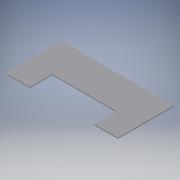
# Autodesk Inventor part: Pared sur
Saved by Autodesk Inventor 2016 (Build 200138000, 138)
## iProperties
Created: 2015-11-12
Part Number: Pared sur
Material: Generic
Document SubType Name: Modeling
Designer: serge
Density: 1 g/cm^3
Mass: 1.9558e+06 g
Surface Area: 787272 cm^2
Volume: 1.9558e+06 cm^3
Appearance: Valor por defecto
Author: serge
Autodesk Inventor part; units mm, degrees
ref_plane "YZ Plane" through (0, 0, 0) normal (1, 0, 0) x (0, 1, 0)
ref_plane "XZ Plane" through (0, 0, 0) normal (0, 1, 0) x (-1, 0, 0)
ref_plane "XY Plane" through (0, 0, 0) normal (0, 0, 1) x (1, 0, 0)
sketch "Sketch1" plane through (0, 0, 0) normal (0, 0, 1) x (1, 0, 0)
  line L0 (-4279.0972, -2988.6181) -> (20.9028, -2988.6181)
  line L1 (20.9028, -2988.6181) -> (20.9028, 11.3819)
  line L2 (20.9028, 11.3819) -> (-4279.0972, 11.3819)
  line L3 (-4279.0972, 11.3819) -> (-4279.0972, -2988.6181)
  point P0 (0, 0)
  dimension "Ancho" = 4300
  dimension "Alto" = 3000
  constraints: 8 end point, 2 parallel, 1 horizontal, 1 perpendicular
  measures "Ancho" distance of L1.end L2.end
  measures "Alto" distance of L0.end L1.end
extrude "Extrusion1" add sketch "Sketch1" along normal blind 50.8
sketch "Sketch2" plane through (0, 0, 50.8) normal (0, 0, 1) x (1, 0, 0)
  line L0 (-4279.0972, -2988.6181) -> (20.9028, -2988.6181) projected
  line L1 (-3579.0972, -988.6181) -> (-679.0972, -988.6181)
  line L2 (-679.0972, -988.6181) -> (-679.0972, -2988.6181)
  line L3 (-679.0972, -2988.6181) -> (-3579.0972, -2988.6181)
  line L4 (-3579.0972, -2988.6181) -> (-3579.0972, -988.6181)
  line L5 (-3579.0972, -988.6181) -> (-679.0972, -2988.6181) construction
  line L6 (-679.0972, -988.6181) -> (-3579.0972, -2988.6181) construction
  line L7 (-4279.0972, 11.3819) -> (-4279.0972, -2988.6181) projected
  point P0 (0, 0)
  point P1 (-2129.0972, -1988.6181)
  dimension "Distanciapuerta" = 2900
  dimension "Alturapuerta" = 2000
  dimension "d10" = 700
  constraints: 12 end point, 2 midpoint, 2 parallel, 1 horizontal, 1 perpendicular, 1 point on line
  measures "Distanciapuerta" distance of L1.start L1.end
  measures "Alturapuerta" distance of L1.end L2.end
  measures "d10" distance between parallel lines of L7 L4
extrude "Extrusion2" cut sketch "Sketch2" against normal through all
equation "\"Ancho\" = PL_S"
equation "\"Alto\" = PA_S"
equation "\"Espesor\" = PE_S"
equation "\"Distanciapuerta\" = DP_S"
equation "\"Alturapuerta\" = AP_S"
equation "\"d10\" = -0.5 * DP_S + 0.5 * PL_S"
equation "\"PL_S\" = 4300"
equation "\"PA_S\" = 3000"
equation "\"PE_S\" = 50.8"
equation "\"DP_S\" = 2900"
equation "\"AP_S\" = 2000"
equation "\"PE_N\" = 50.8"
equation "\"PE_EO\" = 50.8"
equation "\"T_E\" = 50.8"
equation "\"lon_ve\" = 512.5"
equation "\"n_a\" = 3"
equation "\"t_a\" = 19.05"
equation "\"d_a\" = 128.125"
equation "\"lon_ho\" = 749"
equation "\"d_bor\" = 59.92"
equation "\"lon_gui\" = 187.25"
equation "\"esp_gui\" = 461.25"
equation "\"lon_ve2\" = 498.475"
equation "\"n_a2\" = 3"
equation "\"t_a2\" = 124.61875"
equation "\"d_a2\" = 124.61875"
equation "\"lon_ho2\" = 933.45"
equation "\"d_bor2\" = 74.676"
equation "\"lon_gui2\" = 233.3625"
equation "\"esp_gui2\" = 448.6275"
equation "\"UE_L\" = 2111"
equation "\"UE_A\" = 1025"
equation "\"UE_AN\" = 749"
equation "\"UC_L\" = 1314.45"
equation "\"UC_A\" = 996.95"
equation "\"UC_AN\" = 933.45"
equation "\"A_ET\" = 35"
equation "\"SEP_NS\" = 0"
equation "\"DSEG\" = 0"
equation "\"AEGEP_NS\" = 0"
equation "\"DNS\" = 749"
body "Solid1"
